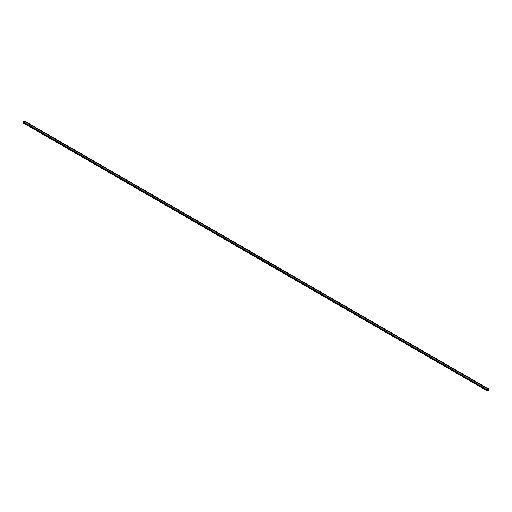
# Autodesk Inventor part: TL20240701-10100CV-RAIL 2
Saved by Autodesk Inventor 2022.5 (Build 265521000, 521)
## iProperties
Category: PROFILE ASSY
Manager: 호상태
Created: 2023-01-20
Part Number: TL20240701-10100CV-RAIL 2
User Status: 1
Material: SS400
Description: 3
Document SubType Name: Modeling
Designer: 박성규
Density: 7.85 g/cm^3
Appearance: 후처리 없음
DETAIL: Coveryor Assembly
M/C TITLE: CJ 제일제당 협동로봇 포장시스탬 PILOT 장비
PARTS NAME: Bracket
SPECIFICATION: TA20221101-CV200000-015
DocNumber: 221118_Standard_v1
Folder: .\
VDS_Category: 엔지니어링
Detail Description: Purchased products
Title: GUIDE B
Author: 박성규
Revision Number: A
Autodesk Inventor part; units mm, degrees
ref_plane "YZ Plane" through (0, 0, 0) normal (1, 0, 0) x (0, 1, 0)
ref_plane "XZ Plane" through (0, 0, 0) normal (0, 1, 0) x (-1, 0, 0)
ref_plane "XY Plane" through (0, 0, 0) normal (0, 0, 1) x (1, 0, 0)
sketch "스케치8" plane through (0, 0, 0) normal (1, 0, 0) x (0, 1, 0)
  line L0 (5, 12.5) -> (-5, 12.5)
  line L1 (-5, 12.5) -> (-5, -12.5)
  line L2 (-5, -12.5) -> (5, -12.5)
  line L3 (5, -12.5) -> (5, 12.5)
  line L4 (5, 12.5) -> (-5, -12.5) construction
  line L5 (-5, 12.5) -> (5, -12.5) construction
  point P0 (0, 0)
  dimension "d38" = 25
  dimension "d39" = 10
  constraints: 12 end point, 2 midpoint, 2 parallel, 1 horizontal, 1 perpendicular
  measures "d38" distance of L2.end L0.start
  measures "d39" distance of L1.end L2.end
extrude "돌출3" add sketch "스케치8" along normal mid plane 7420
